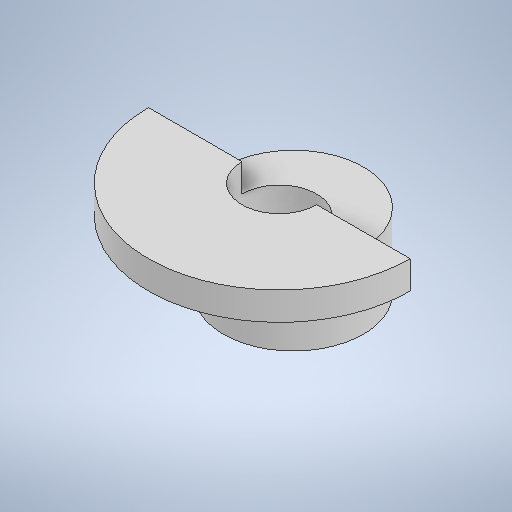
# Autodesk Inventor part: 204
Saved by Autodesk Inventor 2025.1 (Build 291241000, 241)
## iProperties
Created: 2024-08-01
Part Number: 204
Material: Generisch
Document SubType Name: Modeling
Designer: ffogue
Density: 1 g/cm^3
Appearance: Vorgabe
Author: ffogue
Autodesk Inventor part; units mm, degrees
ref_plane "YZ Plane" through (0, 0, 0) normal (1, 0, 0) x (0, 1, 0)
sketch "Sketch1" plane through (0, 0, 0) normal (0, 0, 1) x (1, 0, 0)
  arc A0 (-14, 0) -> (14, 0) centre (0, 0) ccw
  line L0 (-14, 0) -> (14, 0)
  dimension "d0" = 28
  constraints: 2 end point, 2 point on circle, 1 centre point, 1 coincident, 1 horizontal, 1 horizontal alignment, 1 midpoint
  measures "d0" diameter of A0
extrude "Extrusion1" add sketch "Sketch1" along normal blind 3
sketch "Sketch2" plane through (0, 0, 0) normal (0, 0, -1) x (-1, 0, 0)
  circle A0 centre (0, 1.5) radius 7.5
  line L0 (-14, 0) -> (14, 0) projected
  point P0 (0, 0)
  point P1 (0, 0)
  dimension "d22" = 15
  dimension "d23" = 1.5
  constraints: 1 centre point, 1 midpoint, 1 vertical alignment
  measures "d22" diameter of A0
  measures "d23" distance from line of L0 A0.centre
extrude "Extrusion2" add sketch "Sketch2" along normal blind 8
sketch "Sketch3" plane through (0, 0, -8) normal (0, 0, -1) x (-1, 0, 0)
  circle A0 centre (0, 1.5) radius 7.5 projected
  point P0 (0, 0)
  point P1 (0, 0)
  point P2 (0, 0)
  constraints: 2 coincident
hole "Hole1" at (0, 0, -8) direction (0, 0, 1) diameter 8 depth 11
ref_plane "Work Plane1" through (0, 9, 0) normal (0, 1, 0) x (-1, 0, 0)
sketch "Sketch4" plane through (0, 9, 0) normal (0, 1, 0) x (-1, 0, 0)
  line L0 (-7.5, -8) -> (7.5, -8) projected
  line L1 (7.3485, 0) -> (-7.3485, 0) projected
  line L2 (7.3485, 0) -> (-7.3485, 0) projected
  line L3 (7.5, 0) -> (7.5, -8) projected
  line L4 (-7.5, 0) -> (-7.5, -8) projected
  point P0 (0, 0)
  point P1 (0, -4)
  point P2 (0, 0)
  point P3 (-7.5, -4)
  constraints: 1 horizontal alignment, 1 midpoint, 1 vertical alignment
hole "Hole2" at (0, 9, -4) direction (0, -1, 0) diameter 2.459 depth 3.5 thread size "M3x0.5" class "6H" standard "ISO Metric profile"
ref_plane "Work Plane2" through (0, 0, 0) normal (0, 1, 0) x (-1, 0, 0)
mirror "Mirror1" about plane through (0, 0, 0) normal (0, 1, 0) of "Hole2"
body "Solid1"
